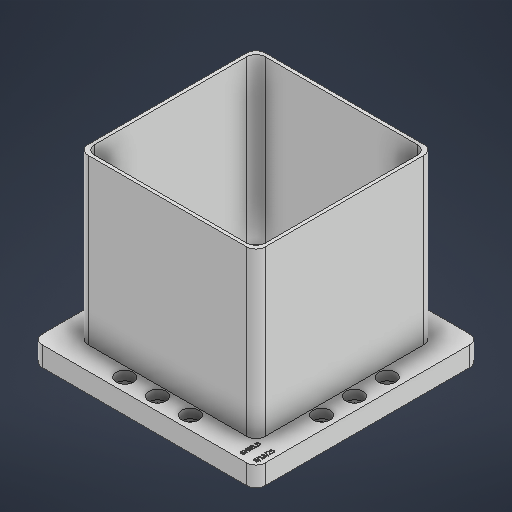
# Autodesk Inventor part: Shield
Saved by Autodesk Inventor 2025 (Build 290162000, 162)
## iProperties
Created: 2025-08-15
Part Number: Shield
Material: Generic
Document SubType Name: Modeling
Designer: mayhem
Density: 1 g/cm^3
Appearance: Default
Author: mayhem
Autodesk Inventor part; units mm, degrees
ref_plane "YZ Plane" through (0, 0, 0) normal (1, 0, 0) x (0, 1, 0)
ref_plane "XZ Plane" through (0, 0, 0) normal (0, 1, 0) x (-1, 0, 0)
ref_plane "XY Plane" through (0, 0, 0) normal (0, 0, 1) x (1, 0, 0)
sketch "Sketch1" plane through (0, 0, 0) normal (0, 1, 0) x (-1, 0, 0)
  line L0 (85, 85) -> (-85, 85)
  line L1 (-85, 85) -> (-85, -85)
  line L2 (-85, -85) -> (85, -85)
  line L3 (85, -85) -> (85, 85)
  line L4 (47, -65) -> (-47, -65)
  line L5 (-65, -47) -> (-65, 47)
  line L6 (-47, 65) -> (47, 65)
  line L7 (65, 47) -> (65, -47)
  line L8 (0, 0) -> (0, 20)
  line L9 (0, 0) -> (15.875, 0)
  arc A0 (-65, -63) -> (-63, -65) centre (-63, -63) ccw
  arc A1 (-65, -47) -> (-47, -65) centre (-47, -47) ccw
  arc A2 (47, -65) -> (65, -47) centre (47, -47) ccw
  arc A3 (65, 47) -> (47, 65) centre (47, 47) ccw
  arc A4 (-47, 65) -> (-65, 47) centre (-47, 47) ccw
  point P0 (65, -65)
  point P1 (-65, -65)
  point P2 (-65, 65)
  point P3 (65, 65)
  point P4 (-65, -45)
  point P5 (-45, -65)
  point P6 (-65, 0)
  point P7 (0, -65)
  dimension "d50" = 45
  dimension "d51" = 170
  dimension "d52" = 170
  dimension "d53" = 20
  dimension "d54" = 130
  dimension "d55" = 130
  dimension "d56" = 45
  dimension "d62" = 2
  dimension "d63" = 20
  dimension "d64" = 18
  constraints: 20 end point, 12 point on line, 10 point on circle, 10 tangent, 5 centre point, 4 parallel, 3 equal radius, 2 midpoint, 2 perpendicular, 1 horizontal, 1 vertical
  measures "d50" distance of point (-65, 0) point (-65, -45)
  measures "d51" distance of L2.end L0.start
  measures "d52" distance of L1.end L2.end
  measures "d53" distance between parallel lines of L2 L4
  measures "d54" distance of point (65, 65) point (65, -65)
  measures "d55" distance of point (65, -65) point (-65, -65)
  measures "d56" distance of point (0, -65) point (-45, -65)
  measures "d62" radius of A0
  measures "d63" distance between parallel lines of L5 L1
  measures "d64" radius of A1
extrude "Extrusion1" add sketch "Sketch1" along normal blind 15
sketch "Sketch3" plane through (0, 15, 0) normal (0, 1, 0) x (1, 0, 0)
  line L0 (-75, 75) -> (75, 75)
  line L1 (75, 75) -> (75, -75)
  line L2 (75, -75) -> (-75, -75)
  line L3 (-75, -75) -> (-75, 75)
  line L4 (-75, 75) -> (75, -75) construction
  line L5 (75, 75) -> (-75, -75) construction
  circle A0 centre (0, -75) radius 3
  circle A1 centre (-25, -75) radius 3
  circle A2 centre (25, -75) radius 3
  circle A3 centre (75, 0) radius 3
  circle A4 centre (75, 25) radius 3
  circle A5 centre (75, -25) radius 3
  circle A6 centre (-75, 0) radius 3
  circle A7 centre (-75, -25) radius 3
  circle A8 centre (-75, 25) radius 3
  circle A9 centre (0, 75) radius 3
  circle A10 centre (25, 75) radius 3
  circle A11 centre (-25, 75) radius 3
  point P0 (0, 0)
  dimension "d30" = 150
  dimension "d31" = 150
  dimension "d32" = 6
  dimension "d33" = 6
  dimension "d34" = 6
  dimension "d35" = 6
  dimension "d36" = 6
  dimension "d37" = 6
  dimension "d38" = 25
  dimension "d39" = 25
  dimension "d40" = 25
  dimension "d41" = 25
  constraints: 12 centre point, 12 end point, 6 symmetric about line, 4 midpoint, 4 point on line, 2 parallel, 1 horizontal, 1 perpendicular, 6 other
  measures "d30" distance of L1.end L2.end
  measures "d31" distance of L0.end L1.end
  measures "d32" diameter of A0
  measures "d33" diameter of A1
  measures "d34" diameter of A2
  measures "d35" diameter of A3
  measures "d36" diameter of A4
  measures "d37" diameter of A5
  measures "d38" distance of A2.centre A0.centre
  measures "d39" distance of A0.centre A1.centre
  measures "d40" distance of A3.centre A5.centre
  measures "d41" distance of A3.centre A4.centre
hole "Hole1" at (-25, 15, 75) at (0, 15, 75) at (25, 15, 75) at (75, 15, 25) at (75, 15, 0) at (75, 15, -25) at (25, 15, -75) at (0, 15, -75) at (-25, 15, -75) at (-75, 15, -25) at (-75, 15, 0) at (-75, 15, 25) direction (0, -1, 0) diameter 7.125 end through all counterbore diameter 13 counterbore depth 7
sketch "Sketch4" plane through (0, 15, 0) normal (0, 1, 0) x (1, 0, 0)
  line L0 (65, 65) -> (-65, 65)
  line L1 (-65, 65) -> (-65, -65)
  line L2 (-65, -65) -> (65, -65)
  line L3 (65, -65) -> (65, 65)
  line L4 (65, 65) -> (-65, -65) construction
  line L5 (-65, 65) -> (65, -65) construction
  line L6 (-67.5, 67.5) -> (67.5, 67.5)
  line L7 (67.5, 67.5) -> (67.5, -67.5)
  line L8 (67.5, -67.5) -> (-67.5, -67.5)
  line L9 (-67.5, -67.5) -> (-67.5, 67.5)
  point P0 (0, 0)
  dimension "d57" = 130
  dimension "d58" = 130
  dimension "d59" = 2.5
  constraints: 20 end point, 4 parallel, 2 midpoint, 2 perpendicular, 1 horizontal, 3 other
  measures "d57" distance of L2.end L1.end
  measures "d58" distance between parallel lines of L0 L2
  measures "d59" distance between parallel lines of L0 L6
extrude "Extrusion3" add sketch "Sketch4" along normal blind 125
fillet "Fillet2" radius 7.125 12 edges at (65, 77.5, 65) (67.5, 77.5, 67.5) (-67.5, 77.5, 67.5) (-65, 77.5, 65) (-65, 77.5, -65) (-67.5, 77.5, -67.5) (67.5, 77.5, -67.5) (65, 77.5, -65) (-85, 7.5, 85) (85, 7.5, 85) (85, 7.5, -85) (-85, 7.5, -85)
sketch "Sketch5" plane through (67.5, 15, 60.375) normal (0, 1, 0) x (0, 0, -1)
  line L0 (-20.576, -0.6389) -> (31.3928, -0.6389) construction
  line L1 (31.3928, -0.6389) -> (31.3928, -37.096) construction
  line L2 (31.3928, -37.096) -> (-20.576, -37.096) construction
  line L3 (-20.576, -37.096) -> (-20.576, -0.6389) construction
  spline S0 degree 2 poles (-19.4176, -3.7956) (-19.7486, -3.7956) (-20.2129, -3.6573) (-20.4179, -3.5585) knots 0 0 0 1 2 2 2
  line L4 (-20.4179, -3.5585) -> (-20.4179, -3.0497)
  line L5 (-20.4179, -3.0497) -> (-20.3883, -3.0497)
  spline S1 degree 2 poles (-20.3883, -3.0497) (-20.1882, -3.2374) (-19.6819, -3.4449) (-19.4472, -3.4449) knots 0 0 0 1 2 2 2
  spline S2 degree 2 poles (-19.4472, -3.4449) (-19.1113, -3.4449) (-18.768, -3.1658) (-18.768, -2.936) knots 0 0 0 1 2 2 2
  spline S3 degree 2 poles (-18.768, -2.936) (-18.768, -2.7533) (-18.9483, -2.526) (-19.1434, -2.4692) knots 0 0 0 1 2 2 2
  spline S4 degree 2 poles (-19.1434, -2.4692) (-19.2842, -2.4297) (-19.5189, -2.3753) (-19.6942, -2.3309) knots 0 0 0 1 2 2 2
  spline S5 degree 2 poles (-19.6942, -2.3309) (-19.8523, -2.2889) (-20.1018, -2.1629) (-20.1981, -2.0617) knots 0 0 0 1 2 2 2
  spline S6 degree 2 poles (-20.1981, -2.0617) (-20.292, -1.9604) (-20.3957, -1.6887) (-20.3957, -1.5108) knots 0 0 0 1 2 2 2
  spline S7 degree 2 poles (-20.3957, -1.5108) (-20.3957, -1.1403) (-19.8177, -0.6389) (-19.3707, -0.6389) knots 0 0 0 1 2 2 2
  spline S8 degree 2 poles (-19.3707, -0.6389) (-19.1138, -0.6389) (-18.6593, -0.7402) (-18.4642, -0.8365) knots 0 0 0 1 2 2 2
  line L6 (-18.4642, -0.8365) -> (-18.4642, -1.3206)
  line L7 (-18.4642, -1.3206) -> (-18.4938, -1.3206)
  spline S9 degree 2 poles (-18.4938, -1.3206) (-18.6395, -1.1873) (-19.094, -0.9897) (-19.3435, -0.9897) knots 0 0 0 1 2 2 2
  spline S10 degree 2 poles (-19.3435, -0.9897) (-19.6251, -0.9897) (-19.9733, -1.254) (-19.9733, -1.4688) knots 0 0 0 1 2 2 2
  spline S11 degree 2 poles (-19.9733, -1.4688) (-19.9733, -1.6615) (-19.7683, -1.8912) (-19.5757, -1.9431) knots 0 0 0 1 2 2 2
  spline S12 degree 2 poles (-19.5757, -1.9431) (-19.4472, -1.9777) (-19.0742, -2.0666) (-18.9507, -2.1036) knots 0 0 0 1 2 2 2
  spline S13 degree 2 poles (-18.9507, -2.1036) (-18.6371, -2.2) (-18.3456, -2.5878) (-18.3456, -2.8718) knots 0 0 0 1 2 2 2
  spline S14 degree 2 poles (-18.3456, -2.8718) (-18.3456, -3.0521) (-18.4913, -3.3979) (-18.6222, -3.519) knots 0 0 0 1 2 2 2
  spline S15 degree 2 poles (-18.6222, -3.519) (-18.768, -3.6523) (-19.1385, -3.7956) (-19.4176, -3.7956) knots 0 0 0 1 2 2 2
  line L8 (-15.72, -3.7413) -> (-16.125, -3.7413)
  line L9 (-16.125, -3.7413) -> (-16.125, -2.2494)
  line L10 (-16.125, -2.2494) -> (-17.528, -2.2494)
  line L11 (-17.528, -2.2494) -> (-17.528, -3.7413)
  line L12 (-17.528, -3.7413) -> (-17.9331, -3.7413)
  line L13 (-17.9331, -3.7413) -> (-17.9331, -0.6933)
  line L14 (-17.9331, -0.6933) -> (-17.528, -0.6933)
  line L15 (-17.528, -0.6933) -> (-17.528, -1.8888)
  line L16 (-17.528, -1.8888) -> (-16.125, -1.8888)
  line L17 (-16.125, -1.8888) -> (-16.125, -0.6933)
  line L18 (-16.125, -0.6933) -> (-15.72, -0.6933)
  line L19 (-15.72, -0.6933) -> (-15.72, -3.7413)
  line L20 (-14.0404, -3.7413) -> (-15.221, -3.7413)
  line L21 (-15.221, -3.7413) -> (-15.221, -3.43)
  line L22 (-15.221, -3.43) -> (-14.8332, -3.43)
  line L23 (-14.8332, -3.43) -> (-14.8332, -1.0045)
  line L24 (-14.8332, -1.0045) -> (-15.221, -1.0045)
  line L25 (-15.221, -1.0045) -> (-15.221, -0.6933)
  line L26 (-15.221, -0.6933) -> (-14.0404, -0.6933)
  line L27 (-14.0404, -0.6933) -> (-14.0404, -1.0045)
  line L28 (-14.0404, -1.0045) -> (-14.4281, -1.0045)
  line L29 (-14.4281, -1.0045) -> (-14.4281, -3.43)
  line L30 (-14.4281, -3.43) -> (-14.0404, -3.43)
  line L31 (-14.0404, -3.43) -> (-14.0404, -3.7413)
  line L32 (-13.5389, -3.7413) -> (-13.5389, -0.6933)
  line L33 (-13.5389, -0.6933) -> (-11.6321, -0.6933)
  line L34 (-11.6321, -0.6933) -> (-11.6321, -1.0539)
  line L35 (-11.6321, -1.0539) -> (-13.1339, -1.0539)
  line L36 (-13.1339, -1.0539) -> (-13.1339, -1.8888)
  line L37 (-13.1339, -1.8888) -> (-11.7334, -1.8888)
  line L38 (-11.7334, -1.8888) -> (-11.7334, -2.2494)
  line L39 (-11.7334, -2.2494) -> (-13.1339, -2.2494)
  line L40 (-13.1339, -2.2494) -> (-13.1339, -3.3806)
  line L41 (-13.1339, -3.3806) -> (-11.6321, -3.3806)
  line L42 (-11.6321, -3.3806) -> (-11.6321, -3.7413)
  line L43 (-11.6321, -3.7413) -> (-13.5389, -3.7413)
  line L44 (-9.4214, -3.7413) -> (-11.1875, -3.7413)
  line L45 (-11.1875, -3.7413) -> (-11.1875, -0.6933)
  line L46 (-11.1875, -0.6933) -> (-10.7824, -0.6933)
  line L47 (-10.7824, -0.6933) -> (-10.7824, -3.3806)
  line L48 (-10.7824, -3.3806) -> (-9.4214, -3.3806)
  line L49 (-9.4214, -3.3806) -> (-9.4214, -3.7413)
  spline S16 degree 2 poles (-6.6995, -2.2197) (-6.6995, -2.6372) (-7.0379, -3.309) (-7.3219, -3.4967) knots 0 0 0 1 2 2 2
  spline S17 degree 2 poles (-7.3219, -3.4967) (-7.5541, -3.6425) (-8.0308, -3.7413) (-8.4013, -3.7413) knots 0 0 0 1 2 2 2
  line L50 (-8.4013, -3.7413) -> (-9.1028, -3.7413)
  line L51 (-9.1028, -3.7413) -> (-9.1028, -0.6933)
  line L52 (-9.1028, -0.6933) -> (-8.4087, -0.6933)
  spline S18 degree 2 poles (-8.4087, -0.6933) (-7.9789, -0.6933) (-7.4899, -0.8217) (-7.317, -0.9353) knots 0 0 0 1 2 2 2
  spline S19 degree 2 poles (-7.317, -0.9353) (-7.023, -1.1305) (-6.6995, -1.7751) (-6.6995, -2.2197) knots 0 0 0 1 2 2 2
  spline S20 degree 2 poles (-7.1218, -2.2148) (-7.1218, -1.8641) (-7.354, -1.3676) (-7.5837, -1.2268) knots 0 0 0 1 2 2 2
  spline S21 degree 2 poles (-7.5837, -1.2268) (-7.7468, -1.1305) (-8.1148, -1.044) (-8.389, -1.044) knots 0 0 0 1 2 2 2
  line L53 (-8.389, -1.044) -> (-8.6977, -1.044)
  line L54 (-8.6977, -1.044) -> (-8.6977, -3.3905)
  line L55 (-8.6977, -3.3905) -> (-8.389, -3.3905)
  spline S22 degree 2 poles (-8.389, -3.3905) (-8.1197, -3.3905) (-7.7122, -3.3041) (-7.5467, -3.188) knots 0 0 0 1 2 2 2
  spline S23 degree 2 poles (-7.5467, -3.188) (-7.3343, -3.0447) (-7.1218, -2.5705) (-7.1218, -2.2148) knots 0 0 0 1 2 2 2
  spline S24 degree 2 poles (-19.4324, -13.8473) (-19.6596, -13.8473) (-20.0326, -13.7115) (-20.1635, -13.5855) knots 0 0 0 1 2 2 2
  spline S25 degree 2 poles (-20.1635, -13.5855) (-20.292, -13.462) (-20.4253, -13.1261) (-20.4253, -12.9359) knots 0 0 0 1 2 2 2
  spline S26 degree 2 poles (-20.4253, -12.9359) (-20.4253, -12.6889) (-20.1611, -12.2739) (-19.9091, -12.1504) knots 0 0 0 1 2 2 2
  line L56 (-19.9091, -12.1504) -> (-19.9091, -12.1381)
  spline S27 degree 2 poles (-19.9091, -12.1381) (-20.1339, -12.0072) (-20.3512, -11.6959) (-20.3512, -11.4638) knots 0 0 0 1 2 2 2
  spline S28 degree 2 poles (-20.3512, -11.4638) (-20.3512, -11.1204) (-19.8325, -10.661) (-19.4324, -10.661) knots 0 0 0 1 2 2 2
  spline S29 degree 2 poles (-19.4324, -10.661) (-19.0174, -10.661) (-18.516, -11.0957) (-18.516, -11.4366) knots 0 0 0 1 2 2 2
  spline S30 degree 2 poles (-18.516, -11.4366) (-18.516, -11.6416) (-18.7556, -12.0417) (-18.9804, -12.1554) knots 0 0 0 1 2 2 2
  line L57 (-18.9804, -12.1554) -> (-18.9804, -12.1677)
  spline S31 degree 2 poles (-18.9804, -12.1677) (-18.7136, -12.2912) (-18.4395, -12.6469) (-18.4395, -12.9285) knots 0 0 0 1 2 2 2
  spline S32 degree 2 poles (-18.4395, -12.9285) (-18.4395, -13.3187) (-19.0076, -13.8473) (-19.4324, -13.8473) knots 0 0 0 1 2 2 2
  spline S33 degree 2 poles (-18.8594, -12.968) (-18.8594, -12.7803) (-19.0076, -12.558) (-19.2175, -12.4444) knots 0 0 0 1 2 2 2
  spline S34 degree 2 poles (-19.2175, -12.4444) (-19.2867, -12.4048) (-19.5189, -12.3134) (-19.6646, -12.2542) knots 0 0 0 1 2 2 2
  spline S35 degree 2 poles (-19.6646, -12.2542) (-19.8325, -12.3653) (-20.0129, -12.6963) (-20.0129, -12.9063) knots 0 0 0 1 2 2 2
  spline S36 degree 2 poles (-20.0129, -12.9063) (-20.0129, -13.1829) (-19.6794, -13.5435) (-19.4275, -13.5435) knots 0 0 0 1 2 2 2
  spline S37 degree 2 poles (-19.4275, -13.5435) (-19.1706, -13.5435) (-18.8594, -13.2348) (-18.8594, -12.968) knots 0 0 0 1 2 2 2
  spline S38 degree 2 poles (-18.9162, -11.4415) (-18.9162, -11.2365) (-19.1903, -10.9623) (-19.4349, -10.9623) knots 0 0 0 1 2 2 2
  spline S39 degree 2 poles (-19.4349, -10.9623) (-19.6572, -10.9623) (-19.9412, -11.2069) (-19.9412, -11.4168) knots 0 0 0 1 2 2 2
  spline S40 degree 2 poles (-19.9412, -11.4168) (-19.9412, -11.5675) (-19.7955, -11.7775) (-19.6498, -11.8614) knots 0 0 0 1 2 2 2
  spline S41 degree 2 poles (-19.6498, -11.8614) (-19.588, -11.896) (-19.3262, -12.017) (-19.22, -12.0516) knots 0 0 0 1 2 2 2
  spline S42 degree 2 poles (-19.22, -12.0516) (-19.0421, -11.9158) (-18.9162, -11.6268) (-18.9162, -11.4415) knots 0 0 0 1 2 2 2
  line L58 (-16.7994, -10.5943) -> (-17.9924, -14.4401)
  line L59 (-17.9924, -14.4401) -> (-18.3382, -14.4401)
  line L60 (-18.3382, -14.4401) -> (-17.1501, -10.5943)
  line L61 (-17.1501, -10.5943) -> (-16.7994, -10.5943)
  line L62 (-14.7369, -13.7782) -> (-16.2239, -13.7782)
  line L63 (-16.2239, -13.7782) -> (-16.2239, -13.4669)
  line L64 (-16.2239, -13.4669) -> (-15.6706, -13.4669)
  line L65 (-15.6706, -13.4669) -> (-15.6706, -11.4242)
  line L66 (-15.6706, -11.4242) -> (-16.2239, -11.4242)
  line L67 (-16.2239, -11.4242) -> (-16.2239, -11.1451)
  spline S43 degree 2 poles (-16.2239, -11.1451) (-15.9102, -11.1451) (-15.6138, -10.9673) (-15.594, -10.7203) knots 0 0 0 1 2 2 2
  line L68 (-15.594, -10.7203) -> (-15.2778, -10.7203)
  line L69 (-15.2778, -10.7203) -> (-15.2778, -13.4669)
  line L70 (-15.2778, -13.4669) -> (-14.7369, -13.4669)
  line L71 (-14.7369, -13.4669) -> (-14.7369, -13.7782)
  spline S44 degree 2 poles (-13.2549, -13.8473) (-13.4821, -13.8473) (-13.8551, -13.7115) (-13.986, -13.5855) knots 0 0 0 1 2 2 2
  spline S45 degree 2 poles (-13.986, -13.5855) (-14.1145, -13.462) (-14.2478, -13.1261) (-14.2478, -12.9359) knots 0 0 0 1 2 2 2
  spline S46 degree 2 poles (-14.2478, -12.9359) (-14.2478, -12.6889) (-13.9835, -12.2739) (-13.7316, -12.1504) knots 0 0 0 1 2 2 2
  line L72 (-13.7316, -12.1504) -> (-13.7316, -12.1381)
  spline S47 degree 2 poles (-13.7316, -12.1381) (-13.9564, -12.0072) (-14.1737, -11.6959) (-14.1737, -11.4638) knots 0 0 0 1 2 2 2
  spline S48 degree 2 poles (-14.1737, -11.4638) (-14.1737, -11.1204) (-13.655, -10.661) (-13.2549, -10.661) knots 0 0 0 1 2 2 2
  spline S49 degree 2 poles (-13.2549, -10.661) (-12.8399, -10.661) (-12.3385, -11.0957) (-12.3385, -11.4366) knots 0 0 0 1 2 2 2
  spline S50 degree 2 poles (-12.3385, -11.4366) (-12.3385, -11.6416) (-12.5781, -12.0417) (-12.8029, -12.1554) knots 0 0 0 1 2 2 2
  line L73 (-12.8029, -12.1554) -> (-12.8029, -12.1677)
  spline S51 degree 2 poles (-12.8029, -12.1677) (-12.5361, -12.2912) (-12.2619, -12.6469) (-12.2619, -12.9285) knots 0 0 0 1 2 2 2
  spline S52 degree 2 poles (-12.2619, -12.9285) (-12.2619, -13.3187) (-12.83, -13.8473) (-13.2549, -13.8473) knots 0 0 0 1 2 2 2
  spline S53 degree 2 poles (-12.6818, -12.968) (-12.6818, -12.7803) (-12.83, -12.558) (-13.04, -12.4444) knots 0 0 0 1 2 2 2
  spline S54 degree 2 poles (-13.04, -12.4444) (-13.1092, -12.4048) (-13.3413, -12.3134) (-13.4871, -12.2542) knots 0 0 0 1 2 2 2
  spline S55 degree 2 poles (-13.4871, -12.2542) (-13.655, -12.3653) (-13.8353, -12.6963) (-13.8353, -12.9063) knots 0 0 0 1 2 2 2
  spline S56 degree 2 poles (-13.8353, -12.9063) (-13.8353, -13.1829) (-13.5019, -13.5435) (-13.25, -13.5435) knots 0 0 0 1 2 2 2
  spline S57 degree 2 poles (-13.25, -13.5435) (-12.9931, -13.5435) (-12.6818, -13.2348) (-12.6818, -12.968) knots 0 0 0 1 2 2 2
  spline S58 degree 2 poles (-12.7387, -11.4415) (-12.7387, -11.2365) (-13.0128, -10.9623) (-13.2574, -10.9623) knots 0 0 0 1 2 2 2
  spline S59 degree 2 poles (-13.2574, -10.9623) (-13.4797, -10.9623) (-13.7637, -11.2069) (-13.7637, -11.4168) knots 0 0 0 1 2 2 2
  spline S60 degree 2 poles (-13.7637, -11.4168) (-13.7637, -11.5675) (-13.618, -11.7775) (-13.4723, -11.8614) knots 0 0 0 1 2 2 2
  spline S61 degree 2 poles (-13.4723, -11.8614) (-13.4105, -11.896) (-13.1487, -12.017) (-13.0425, -12.0516) knots 0 0 0 1 2 2 2
  spline S62 degree 2 poles (-13.0425, -12.0516) (-12.8646, -11.9158) (-12.7387, -11.6268) (-12.7387, -11.4415) knots 0 0 0 1 2 2 2
  line L74 (-10.6219, -10.5943) -> (-11.8149, -14.4401)
  line L75 (-11.8149, -14.4401) -> (-12.1607, -14.4401)
  line L76 (-12.1607, -14.4401) -> (-10.9726, -10.5943)
  line L77 (-10.9726, -10.5943) -> (-10.6219, -10.5943)
  line L78 (-8.4062, -13.7782) -> (-10.2859, -13.7782)
  line L79 (-10.2859, -13.7782) -> (-10.2859, -13.3459)
  spline S63 degree 2 poles (-10.2859, -13.3459) (-10.0834, -13.1557) (-9.7228, -12.8025) (-9.5499, -12.6123) knots 0 0 0 1 2 2 2
  spline S64 degree 2 poles (-9.5499, -12.6123) (-9.2016, -12.2295) (-8.9472, -11.77) (-8.9472, -11.5255) knots 0 0 0 1 2 2 2
  spline S65 degree 2 poles (-8.9472, -11.5255) (-8.9472, -11.3971) (-9.0262, -11.2044) (-9.0979, -11.1427) knots 0 0 0 1 2 2 2
  spline S66 degree 2 poles (-9.0979, -11.1427) (-9.1695, -11.0809) (-9.3572, -11.0192) (-9.4708, -11.0192) knots 0 0 0 1 2 2 2
  spline S67 degree 2 poles (-9.4708, -11.0192) (-9.5795, -11.0192) (-9.8018, -11.0735) (-9.9031, -11.1155) knots 0 0 0 1 2 2 2
  spline S68 degree 2 poles (-9.9031, -11.1155) (-9.9895, -11.1501) (-10.1501, -11.2489) (-10.1995, -11.2835) knots 0 0 0 1 2 2 2
  line L80 (-10.1995, -11.2835) -> (-10.2217, -11.2835)
  line L81 (-10.2217, -11.2835) -> (-10.2217, -10.8487)
  spline S69 degree 2 poles (-10.2217, -10.8487) (-10.0957, -10.787) (-9.6437, -10.6659) (-9.4412, -10.6659) knots 0 0 0 1 2 2 2
  spline S70 degree 2 poles (-9.4412, -10.6659) (-9.0139, -10.6659) (-8.5322, -11.118) (-8.5322, -11.5033) knots 0 0 0 1 2 2 2
  spline S71 degree 2 poles (-8.5322, -11.5033) (-8.5322, -11.6836) (-8.6162, -11.9849) (-8.6903, -12.1134) knots 0 0 0 1 2 2 2
  spline S72 degree 2 poles (-8.6903, -12.1134) (-8.7644, -12.2468) (-8.9793, -12.5086) (-9.0979, -12.6346) knots 0 0 0 1 2 2 2
  spline S73 degree 2 poles (-9.0979, -12.6346) (-9.2905, -12.8445) (-9.7623, -13.294) (-9.9031, -13.425) knots 0 0 0 1 2 2 2
  line L82 (-9.9031, -13.425) -> (-8.4062, -13.425)
  line L83 (-8.4062, -13.425) -> (-8.4062, -13.7782)
  spline S74 degree 2 poles (-6.1511, -12.8099) (-6.1511, -13.0298) (-6.2919, -13.4052) (-6.4204, -13.5435) knots 0 0 0 1 2 2 2
  spline S75 degree 2 poles (-6.4204, -13.5435) (-6.5488, -13.6818) (-6.9316, -13.8424) (-7.1688, -13.8424) knots 0 0 0 1 2 2 2
  spline S76 degree 2 poles (-7.1688, -13.8424) (-7.3861, -13.8424) (-7.811, -13.7461) (-7.9666, -13.6695) knots 0 0 0 1 2 2 2
  line L84 (-7.9666, -13.6695) -> (-7.9666, -13.2372)
  line L85 (-7.9666, -13.2372) -> (-7.9369, -13.2372)
  spline S77 degree 2 poles (-7.9369, -13.2372) (-7.89, -13.2718) (-7.7146, -13.3607) (-7.6084, -13.4003) knots 0 0 0 1 2 2 2
  spline S78 degree 2 poles (-7.6084, -13.4003) (-7.4874, -13.4422) (-7.2873, -13.4892) (-7.1614, -13.4892) knots 0 0 0 1 2 2 2
  spline S79 degree 2 poles (-7.1614, -13.4892) (-7.0379, -13.4892) (-6.8057, -13.4003) (-6.7217, -13.3039) knots 0 0 0 1 2 2 2
  spline S80 degree 2 poles (-6.7217, -13.3039) (-6.6451, -13.2125) (-6.5661, -12.9705) (-6.5661, -12.8075) knots 0 0 0 1 2 2 2
  spline S81 degree 2 poles (-6.5661, -12.8075) (-6.5661, -12.6444) (-6.655, -12.4369) (-6.739, -12.3678) knots 0 0 0 1 2 2 2
  spline S82 degree 2 poles (-6.739, -12.3678) (-6.8254, -12.2912) (-7.0823, -12.227) (-7.2379, -12.227) knots 0 0 0 1 2 2 2
  spline S83 degree 2 poles (-7.2379, -12.227) (-7.4059, -12.227) (-7.7393, -12.2789) (-7.8406, -12.3011) knots 0 0 0 1 2 2 2
  line L86 (-7.8406, -12.3011) -> (-7.8406, -10.7302)
  line L87 (-7.8406, -10.7302) -> (-6.1684, -10.7302)
  line L88 (-6.1684, -10.7302) -> (-6.1684, -11.0883)
  line L89 (-6.1684, -11.0883) -> (-7.4479, -11.0883)
  line L90 (-7.4479, -11.0883) -> (-7.4479, -11.901)
  spline S84 degree 2 poles (-7.4479, -11.901) (-7.3738, -11.8911) (-7.2305, -11.8837) (-7.1712, -11.8837) knots 0 0 0 1 2 2 2
  spline S85 degree 2 poles (-7.1712, -11.8837) (-6.9366, -11.8837) (-6.613, -11.9602) (-6.4648, -12.0739) knots 0 0 0 1 2 2 2
  spline S86 degree 2 poles (-6.4648, -12.0739) (-6.3141, -12.1875) (-6.1511, -12.5333) (-6.1511, -12.8099) knots 0 0 0 1 2 2 2
  point P0 (60.375, 67.5)
  constraints: 2 other
extrude "Extrusion4" cut sketch "Sketch5" against normal blind 3
body "Solid1"
